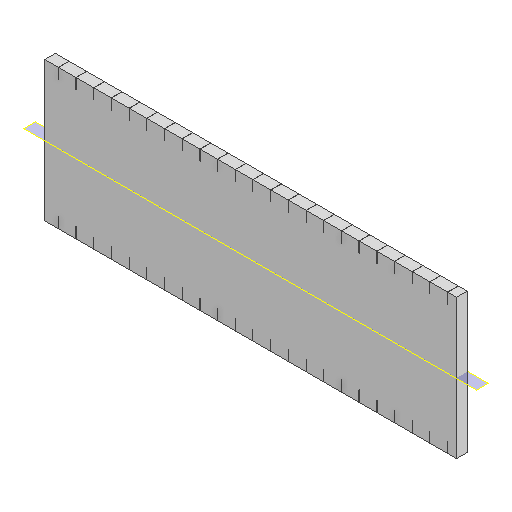
# Autodesk Inventor part: 00_Baseplate_Simmo_side3_v2
Saved by Autodesk Inventor 2022 (Build 260153000, 153)
## iProperties
Created: 2022-08-04
Part Number: 00_Baseplate_Simmo_side3_v2
Material: Generic
Document SubType Name: Modeling
Designer: wanghaoran
Density: 1 g/cm^3
Appearance: Default
Author: wanghaoran
Autodesk Inventor part; units mm, degrees
ref_plane "YZ Plane" through (0, 0, 0) normal (1, 0, 0) x (0, 1, 0)
ref_plane "XZ Plane" through (0, 0, 0) normal (0, 1, 0) x (-1, 0, 0)
ref_plane "XY Plane" through (0, 0, 0) normal (0, 0, 1) x (1, 0, 0)
sketch "Sketch3" plane through (0, 0, 0) normal (0, 0, 1) x (1, 0, 0)
  line L0 (0.8003, 0) -> (0.8003, 6) projected
  line L1 (0.8003, 0) -> (0.8003, -73) projected
  line L2 (-244.2385, 0) -> (-244.2385, 6) projected
  line L3 (0.8003, 6) -> (-231.8779, 6)
  line L4 (-231.8779, 6) -> (-231.8779, -73)
  line L5 (-231.8779, -73) -> (0.8003, -73)
  line L6 (0.8003, -73) -> (0.8003, 6)
  point P0 (0, 0)
  point P1 (-231.8779, 0)
  dimension "d10" = 79
  constraints: 8 end point, 2 parallel, 1 horizontal, 1 perpendicular
  measures "d10" distance of L4.end L3.end
extrude "Extrusion3" add sketch "Sketch3" along normal blind 6
sketch "Sketch4" plane through (0, 0, 6) normal (0, 0, 1) x (1, 0, 0)
  line L0 (0.8003, 6) -> (-231.8779, 6) projected
  line L1 (-234.2385, 6) -> (-234.2385, 0) projected
  line L2 (-224.2385, 0) -> (-224.2385, 6) projected
  line L3 (-234.2385, 0) -> (-224.2385, 0) projected
  line L4 (-224.2385, 6) -> (-224.1385, 6)
  line L5 (-224.1385, 6) -> (-224.1385, 0)
  line L6 (-224.1385, 0) -> (-224.2385, 0)
  line L7 (-224.2385, 0) -> (-224.2385, 6)
  line L8 (-234.2385, 6) -> (-234.3385, 6)
  line L9 (-234.3385, 6) -> (-234.3385, 0)
  line L10 (-234.3385, 0) -> (-234.2385, 0)
  line L11 (-234.2385, 0) -> (-234.2385, 6)
  point P0 (0, 0)
  point P1 (-221.9779, 6)
  point P2 (-224.2385, 0)
  point P3 (-221.8779, 1.1459)
  point P4 (-221.9779, 1.0974)
  point P5 (-221.9779, 5.9515)
  point P6 (-224.2385, 4.8541)
  dimension "d15" = 0.1
  dimension "d16" = 0.1
  constraints: 16 end point, 4 parallel, 2 horizontal, 2 perpendicular, 1 point on line
  measures "d15" distance of L5.end L6.end
  measures "d16" distance of L10.end L9.end
extrude "Extrusion4" cut sketch "Sketch4" against normal blind 6
pattern_linear "Rectangular Pattern2" count 12 spacing 20 along (1, 0, 0) of "Extrusion4"
ref_plane "Work Plane2" through (-231.8779, -33.5, 0) normal (0, -1, 0) x (1, 0, 0)
mirror "Mirror2" about plane through (-231.8779, -33.5, 0) normal (0, -1, 0) of "Extrusion4", "Rectangular Pattern2"
body "Solid2"
